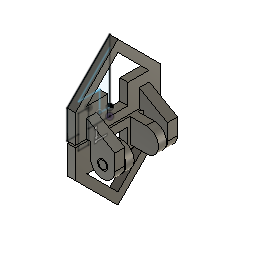
3D프린터 운용기능사 공개도면9 (Autodesk Fusion 360 design; units mm, degrees)
Autodesk Fusion 360 part; units mm, degrees
sketch "Sketch1" plane through (0, 0, 0) normal (1, 0, 0) x (0, 1, 0)
  line L0 (0, 0) -> (0, 35)
  line L1 (-21, 0) -> (-21, 14)
  line L2 (-15.3431, 14) -> (-5, 14)
  line L3 (-21, 14) -> (0, 35)
  line L4 (-15.3431, 14) -> (0, 29.3431)
  line L5 (-5, 4) -> (0, 4)
  line L6 (-5, 4) -> (-5, 14)
  line L7 (-15.5, 9) -> (-15.5, 0)
  line L8 (-10.5, 9) -> (-10.5, 0)
  line L9 (-15.5, 9) -> (-10.5, 9)
  line L10 (0, 0) -> (-10.5, 0)
  line L11 (-15.5, 0) -> (-21, 0)
  line L12 (-15.5, 0) -> (-15.5, -7)
  line L13 (-15.5, -7) -> (-10.5, -7)
  line L14 (-10.5, -7) -> (-10.5, 0)
  point P0 (0, 4)
  point P1 (-5, 4)
  dimension "d1" = 35
  dimension "d2" = 21
  dimension "d3" = 14
  dimension "d5" = 4
  dimension "d6" = 5
  dimension "d7" = 9
  dimension "d8" = -5
  dimension "d9" = 7
  dimension "d49" = 10.5
  constraint vertical L0
  constraint coincident L0.start L10.start
  constraint perpendicular L0 L10
  constraint perpendicular L1 L10
  constraint perpendicular L0 L2
  constraint parallel L3 L4
  constraint coincident L0 P0
  constraint coincident P1 L5.start
  constraint perpendicular L0 L5
  constraint perpendicular L2 L6
  constraint coincident L0 L4.end
  constraint perpendicular L2 L7
  constraint coincident L7.end L10
  constraint coincident L7.start L9.start
  constraint coincident L8 L9.end
  constraint perpendicular L8 L9
  constraint collinear L10 L11
  constraint perpendicular L11 L12
  constraint perpendicular L8 L13
  constraint perpendicular L10 L14
  measures "d1" distance of L0.start L0.end
  measures "d2" distance of L0.start L1.start
  measures "d3" distance of L1.start L1.end
  measures "d5" distance of L0.start P0
  measures "d6" distance of P0 P1
  measures "d7" distance of L7.end L7.start
  measures "d9" distance of L7.end L12.end
  measures "d49" distance of L0 L8
extrude "Extrude1" add sketch "Sketch1" along normal blind 4 contours L0 L1 L2 L3 L4 L5 L6 L7 L8 L9 L10 L11 makes body 1
extrude "Extrude2" add sketch "Sketch1" along normal blind 4 contours L7 L8 L9 L12 L13 L14 bodies 1
extrude "Extrude3" add sketch "Sketch1" along normal blind 14 from surface at 4 contours L7 L8 L9 L12 L13 L14 bodies 1
sketch "Sketch2" plane through (0, -10.5, 0) normal (0, 1, 0) x (-1, 0, 0)
  line L0 (0, 0) -> (-4, 0)
  line L1 (-4, 0) -> (-4, 9)
  line L2 (-4, 9) -> (-18, 9)
  line L3 (-18, 9) -> (-18, -7)
  line L4 (-18, -7) -> (0, -7)
  line L5 (0, -7) -> (0, 0)
  line L6 (-18, 1) -> (-4, 9)
  line L7 (-6, -7) -> (-6, 0)
  line L8 (-6, 0) -> (0, 0)
  line L9 (-18, -7) -> (-6, -7)
  circle A0 centre (-12, -7) radius 2
  arc A1 (-18, -7) -> (-6, -7) centre (-12, -7) ccw
  point P0 (-18, 1)
  point P1 (0, -7)
  dimension "d17" = 6
  dimension "d18" = 8
  dimension "d19" = 4
  constraint coincident L3 P0
  constraint coincident L4 L7.start
  constraint coincident P0 L6.start
  constraint coincident L1.end L2.start
  constraint coincident L7.start L9.end
  constraint perpendicular L0 L7
  constraint coincident L0.start L5.end
  constraint perpendicular L5 L8
  constraint coincident L3.end L4.start
  constraint midpoint L9 A0.centre
  constraint concentric A0 A1
  measures "d17" distance of L7.start P1
  measures "d18" distance of L2.end P0
  measures "d19" diameter of A0
extrude "Extrude4" cut sketch "Sketch2" against normal blind 5 contours L0 L4 L5 L7 L8 | L2 L3 L6 | L4 L9 A0 picked at (-11.4527, -6.1579) bodies 1
extrude "Extrude5" add sketch "Sketch2" against normal blind 5 contours L4 L9 A0 A1 bodies 1
mirror "Mirror1" about plane through (0, 0, 29.3431) normal (0, 1, 0) of bodies 1 makes body 2
combine "Combine1" operation add target body 1 tool bodies 2
sketch "Sketch1 (2)" plane through (0, 0, 0) normal (1, 0, 0) x (0, 1, 0) in component "Component"
  line L0 (0, 0) -> (0, 35)
  line L1 (0, 35) -> (-21, 35)
  line L2 (-21, 35) -> (-21, 21)
  line L3 (-21, 21) -> (0, 0)
  line L4 (0, 31) -> (-5, 31)
  line L5 (-15.3431, 21) -> (0, 5.6569)
  line L6 (-5, 31) -> (-5, 21)
  line L7 (-5, 21) -> (-15.3431, 21)
  line L8 (-10, 35) -> (-10, 23)
  line L9 (-6, 35) -> (-6, 23)
  line L10 (-6, 23) -> (-10, 23)
  point P0 (-10, 35)
  dimension "d25" = 35
  dimension "d26" = 21
  dimension "d27" = 14
  dimension "d29" = 4
  dimension "d30" = 5
  dimension "d31" = 10
  dimension "d32" = 10
  dimension "d33" = 12
  dimension "d34" = -4
  constraint coincident L0.start L3.end
  constraint vertical L0
  constraint perpendicular L0 L1
  constraint perpendicular L1 L2
  constraint coincident L0 L4.start
  constraint parallel L1 L4
  constraint parallel L3 L5
  constraint coincident L4.end L6.start
  constraint perpendicular L4 L6
  constraint coincident L0 L5.end
  constraint perpendicular L6 L7
  constraint coincident L1 P0
  constraint coincident P0 L8.start
  constraint perpendicular L1 L8
  constraint perpendicular L8 L10
  measures "d25" distance of L0.start L0.end
  measures "d26" distance of L0.end L1.end
  measures "d27" distance of L1.end L2.end
  measures "d29" distance of L0.end L4.start
  measures "d30" distance of L0 L4.end
  measures "d31" distance of L4.end L6.end
  measures "d32" distance of L0 P0
  measures "d33" distance of P0 L8.end
extrude "Extrude1'" add sketch "Sketch1 (2)" along normal blind 4 separate body contours L0 L1 L2 L3 L4 L5 L6 L7 L8 L9 L10 | L1 L8 L9 L10 makes body 3 in component "Component"
extrude "Extrude2'" add sketch "Sketch1 (2)" along normal blind 12 contours L1 L8 L9 L10 bodies 3 in component "Component"
sketch "Sketch2 (2)" plane through (0, -6, 0) normal (0, 1, 0) x (-1, 0, 0) in component "Component"
  line L0 (-4, 23) -> (-4, 35)
  line L1 (-4, 35) -> (-12, 35)
  line L2 (-12, 35) -> (-12, 23)
  line L3 (-12, 23) -> (-4, 23)
  circle A0 centre (-12, 29) radius 2.5
  arc A1 (-12, 35) -> (-12, 23) centre (-12, 29) ccw
  dimension "d40" = 5
  dimension "d50" = 6
  constraint midpoint L2 A0.centre
  constraint concentric A0 A1
  measures "d40" diameter of A0
  measures "d50" radius of A1
extrude "Extrude3'" add sketch "Sketch2 (2)" against normal blind 4 contours L2 A0 A1 bodies 3 in component "Component"
extrude "Extrude4'" add sketch "Sketch2 (2)" against normal blind 5.5 from surface at -4 separate body contours L2 A0 | L2 A0 makes body 4 in component "Component"
extrude "Extrude5'" add sketch "Sketch2 (2)" against normal blind 9.5 contours L2 A0 picked at (-12.9366, 28.4168) bodies 4 3 in component "Component"
mirror "Mirror1'" about plane through (0, 0, 31) normal (0, 1, 0) of bodies 4 makes body 5 in component "Component"
combine "Combine1'" operation add target body 4 tool bodies 5 in component "Component"
copy_body "Body->Comp1" bodies 1 removing the originals makes body 6 in component "Component'"
component "Component" placed x (1, 0, 0) y (0, 1, 0) z (0, 0, 1) at (0, 0, -36)
component "Component'" placed x (1, 0, 0) y (0, 1, 0) z (0, 0, 1) at (0, 0, 0)
